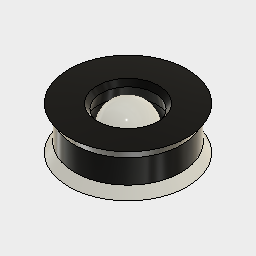
Lens Holder (Autodesk Fusion 360 design; units mm, degrees)
Autodesk Fusion 360 part; units mm, degrees
sketch "Sketch2" plane through (0, 0, 0) normal (0, 0, 1) x (1, 0, 0)
sphere "SpherePrimitive2" add diameter 2 placed x (1, 0, 0) y (0, 1, 0) z (0, 0, 1) at (0, 0, 0) makes body 1
sketch "Sketch3" plane through (0, 0, 0) normal (0, 1, 0) x (1, 0, 0)
  circle A0 centre (0, 0) radius 1.25
  line L0 (-2.5, -0.9) -> (2.5, -0.9)
  line L1 (2.5, -0.9) -> (2.5, 0.9)
  line L2 (2.5, 0.9) -> (-2.5, 0.9)
  line L3 (-2.5, 0.9) -> (-2.5, -0.9)
  line L4 (-1.1, -0.9) -> (-1.2276, -0.2358)
  line L5 (1.1, -0.9) -> (1.2276, -0.2358)
  line L6 (0, -0.9) -> (0, 0.9)
  line L7 (-2.25, -0.5) -> (2.25, -0.5)
  line L8 (2.25, -0.5) -> (2.25, 0.5)
  line L9 (2.25, 0.5) -> (-2.25, 0.5)
  line L10 (-2.25, 0.5) -> (-2.25, -0.5)
  line L11 (2.25, -0.5) -> (2.5, -0.9)
  line L12 (2.25, 0.5) -> (2.5, 0.9)
  dimension "d3" = 2.5
  dimension "d4" = 5
  dimension "d5" = 2.5
  dimension "d6" = 1.8
  dimension "d7" = 0.9
  dimension "d8" = 1.4
  dimension "d9" = 1.4
  dimension "d11" = 4.5
  dimension "d12" = 1
  dimension "d13" = 0.5
  dimension "d14" = 2.25
  measures "d3" diameter of A0
  measures "d4" distance of L0.start L0.end
  measures "d5" distance of A0.centre L3
  measures "d6" distance of L0.start L2.end
  measures "d7" distance of A0.centre L0
  measures "d8" distance of L1 L5.start
  measures "d9" distance of L3 L4.start
  measures "d11" distance of L7.start L7.end
  measures "d12" distance of L7.start L9.end
  measures "d13" distance of A0.centre L7
  measures "d14" distance of A0.centre L8
revolve "Revolve1" add sketch "Sketch3" angle 360 about axis through (0, 0, 0.9) along (0, 0, -1) separate body contours A0 L5 L7 L8 L9 | L0 L5 L7 L11 | A0 L2 L9 L12 makes body 2
chamfer "Chamfer1" distance 0.2 angle 45 1 edges at (-1.0256, -0.3978, 0.9) on bodies 2
ref_plane "WorkPlane1" through (0, 0, -0.5) normal (0, 0, 1) x (1, 0, 0)
split "Split1" by plane through (0, 0, -0.5) normal (0, 0, 1) bodies 2 makes body 3 at (2.0907, 0.1242, 0.9)
equation "d5 = d4 / 2"
equation "d7 = d6 / 2"
equation "d9 = d8"
equation "d13 = d12 / 2"
equation "d14 = d11 / 2"
